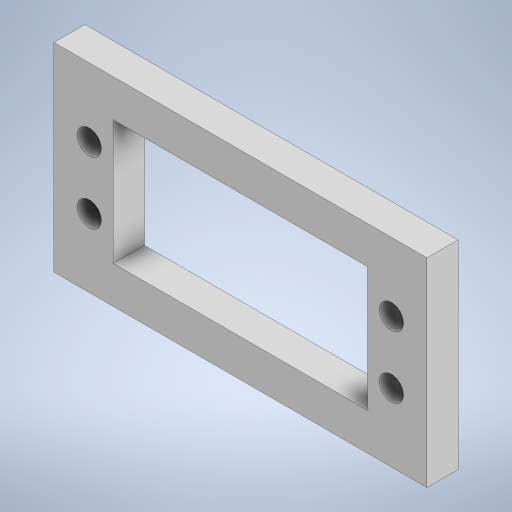
# Autodesk Inventor part: servo_case
Saved by Autodesk Inventor 2024.3 (Build 283343000, 343)
## iProperties
Created: 2024-10-22
Part Number: servo_case
Material: 一般
Document SubType Name: Modeling
Designer: 佐藤智貴
Density: 1 g/cm^3
Appearance: 既定
Author: 佐藤智貴
Autodesk Inventor part; units mm, degrees
ref_plane "YZ Plane" through (0, 0, 0) normal (1, 0, 0) x (0, 1, 0)
ref_plane "XZ Plane" through (0, 0, 0) normal (0, 1, 0) x (-1, 0, 0)
ref_plane "XY Plane" through (0, 0, 0) normal (0, 0, 1) x (1, 0, 0)
sketch "スケッチ2" plane through (0, 0, 0) normal (0, 0, 1) x (1, 0, 0)
  line L0 (0, 0) -> (60, 0)
  line L1 (60, 0) -> (60, 32)
  line L2 (60, 32) -> (0, 32)
  line L3 (0, 32) -> (0, 0)
  line L4 (3, 26) -> (57, 26)
  line L5 (57, 26) -> (57, 6)
  line L6 (57, 6) -> (3, 6)
  line L7 (3, 6) -> (3, 26)
  circle A0 centre (5.7, 21) radius 1.95
  circle A1 centre (5.7, 11) radius 1.95
  circle A2 centre (54.3, 21) radius 1.95
  circle A3 centre (54.3, 11) radius 1.95
  line L8 (9.55, 26) -> (50.45, 26)
  line L9 (50.45, 26) -> (50.45, 6)
  line L10 (50.45, 6) -> (9.55, 6)
  line L11 (9.55, 6) -> (9.55, 26)
  point P0 (30, 0)
  point P1 (9.55, 6)
  dimension "d78" = 20
  dimension "d79" = 3.9
  dimension "d80" = 3.9
  dimension "d81" = 3.9
  dimension "d82" = 3.9
  dimension "d83" = 48.6
  dimension "d84" = 54
  dimension "d85" = 2.7
  dimension "d86" = 2.7
  dimension "d87" = 48.6
  dimension "d88" = 10
  dimension "d89" = 5
  dimension "d90" = 10
  dimension "d91" = 5
  dimension "d92" = 60
  dimension "d93" = 3
  dimension "d94" = 40.9
  dimension "d95" = 6.55
  dimension "d96" = 6.55
  dimension "d97" = 32
  dimension "d98" = 6
  constraints: 24 end point, 6 parallel, 4 centre point, 3 horizontal, 3 perpendicular, 2 point on line, 1 midpoint
  measures "d78" distance between parallel lines of L6 L4
  measures "d79" diameter of A0
  measures "d80" diameter of A1
  measures "d81" diameter of A3
  measures "d82" diameter of A2
  measures "d83" distance of A2.centre A0.centre
  measures "d84" distance of L4.start L4.end
  measures "d85" distance from line of L7 A0.centre
  measures "d86" distance from line of L7 A1.centre
  measures "d87" distance of A1.centre A3.centre
  measures "d88" distance of A1.centre A0.centre
  measures "d89" distance from line of L4 A0.centre
  measures "d90" distance between centres of A2 A3
  measures "d91" distance from line of L4 A2.centre
  measures "d92" distance of L1.end L2.end
  measures "d93" distance between parallel lines of L3 L7
  measures "d94" distance between parallel lines of L9 L11
  measures "d95" distance between parallel lines of L7 L11
  measures "d96" distance between parallel lines of L5 L9
  measures "d97" distance between parallel lines of L0 L2
  measures "d98" distance from line of point (30, 0) L10
extrude "押し出し2" add sketch "スケッチ2" along normal blind 5 contours L3 L2 L1 L0 | L4 L11 L6 L7 | L4 L5 L6 L9
equation "\"d80\" = d79"
equation "\"d81\" = d79"
equation "\"d82\" = d79"
equation "\"d86\" = d85"
equation "\"d87\" = d83"
equation "\"d90\" = d88"
equation "\"d91\" = d89"
